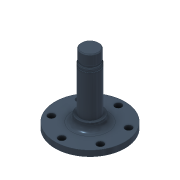
# Autodesk Inventor part: 7055-191 PART1
Saved by Autodesk Inventor 2020.1 (Build 241239000, 239)
## iProperties
Created: 2001-03-07
Part Number: 7055-191 PART1
Document SubType Name: Modeling
Designer: Joe M
Material: Steel, Mild
Engineer: Joe M
Cost Center: 6.680 kg
Authority: 849920.0 mm^3
Density: 7.86 g/cm^3
Appearance: Blue Gray (Dark/Polished)
Control State: 0
Master: False
Checked Out: False
Shininess: 20.0
Length Units: 11269
Angle Units: 11279
Time Units: 11290
Mass Units: 11283
Length Display Precision: 3
Angle Display Precision: 2
Compacted: True
SaveDate: 2003-11-30
SaveTime: 16:18
TotalMass: 6.680 kg
TotalVolume: 849920.0 mm^3
Density: 0.0
Volumn: 0.0
Area: 0.0
PropertySet Name: Model Information
Author: Joe M
Autodesk Inventor part; units mm, degrees
ref_plane "YZ Plane" through (0, 0, 0) normal (1, 0, 0) x (0, 1, 0)
ref_plane "XZ Plane" through (0, 0, 0) normal (0, 1, 0) x (-1, 0, 0)
ref_plane "XY Plane" through (0, 0, 0) normal (0, 0, 1) x (1, 0, 0)
sketch "Sketch1" plane through (-207.0981, -171.1026, -7.5) normal (0, 0, 1) x (1, 0, 0)
  circle A0 centre (207.0981, 171.1026) radius 92.5
  dimension "d40" = 185
  constraints: 1 centre point, 1 other
  measures "d40" diameter of A0
extrude "ExtrusionBlind1" add sketch "Sketch1" along normal blind 15
sketch "Sketch2" plane through (-207.0981, -171.1026, -7.5) normal (0, 0, 1) x (1, 0, 0)
  circle A0 centre (207.0981, 171.1026) radius 57.5
  circle A1 centre (207.0981, 171.1026) radius 92.5 projected
  dimension "d41" = 115
  constraints: 1 centre point, 1 concentric
  measures "d41" diameter of A0
extrude "ExtrusionBlind2" add sketch "Sketch2" against normal blind 10 contours A0
chamfer "Chamfer1" distance 2 angle 30 1 edges at (-57.5, 0, -17.5) measured on face at (-40.0277, -41.2799, -14.1667)
sketch "Sketch4" plane through (0, 0, 7.5) normal (0, 0, 1) x (1, 0, 0)
  circle A0 centre (0, 0) radius 32.5
  circle A1 centre (0, 0) radius 92.5 projected
  dimension "d42" = 65
  constraints: 1 centre point, 1 concentric
  measures "d42" diameter of A0
extrude "ExtrusionBlind3" add sketch "Sketch4" along normal blind 20 contours A0
fillet "Fillet1" radius 15 1 edges at (-32.5, 0, 7.5)
sketch "Sketch5" plane through (0, 0, 27.5) normal (0, 0, 1) x (1, 0, 0)
  circle A0 centre (0, 0) radius 25
  circle A1 centre (0, 0) radius 32.5 projected
  dimension "d43" = 50
  constraints: 3 other
  measures "d43" diameter of A0
extrude "ExtrusionBlind4" add sketch "Sketch5" along normal blind 110 contours A0
sketch "Sketch6" plane through (0, 0, 137.5) normal (0, 0, 1) x (1, 0, 0)
  circle A0 centre (0, 0) radius 23.5
  circle A1 centre (0, 0) radius 25 projected
  dimension "d44" = 47
  constraints: 3 other
  measures "d44" diameter of A0
extrude "ExtrusionBlind5" add sketch "Sketch6" along normal blind 4.15 contours A0
sketch "Sketch7" plane through (0, 0, 141.65) normal (0, 0, 1) x (1, 0, 0)
  circle A0 centre (0, 0) radius 25
  circle A1 centre (0, 0) radius 23.5 projected
  dimension "d45" = 50
  constraints: 3 other
  measures "d45" diameter of A0
extrude "ExtrusionBlind6" add sketch "Sketch7" along normal blind 4.85 contours A0 | A1
chamfer "Chamfer2" distance 2 angle 30 1 edges at (-25, 0, 146.5) measured on face at (24.9189, -2.0117, 144.8833)
sketch "Sketch8" plane through (0, 0, 146.5) normal (0, 0, 1) x (1, 0, 0)
  circle A0 centre (0, 0) radius 21.5
  circle A1 centre (0, 0) radius 23.8453 projected
  dimension "d46" = 43
  constraints: 1 centre point, 1 concentric
  measures "d46" diameter of A0
extrude "ExtrusionBlind7" add sketch "Sketch8" along normal blind 6 contours A0
sketch "Sketch9" plane through (0, 0, 152.5) normal (0, 0, 1) x (1, 0, 0)
  circle A0 centre (0, 0) radius 23.6
  circle A1 centre (0, 0) radius 21.5 projected
  dimension "d47" = 47.2
  constraints: 1 centre point, 1 concentric
  measures "d47" diameter of A0
extrude "ExtrusionBlind8" add sketch "Sketch9" along normal blind 26 contours A0 | A1
chamfer "Chamfer3" distance 2 angle 45 1 edges at (-23.6, 0, 178.5)
sketch "Sketch12" plane through (0, 0, 7.5) normal (0, 0, 1) x (1, 0, 0)
  circle A0 centre (0, 0) radius 92.5 projected
  line L0 (0, 0) -> (0, 75) construction
  dimension "d51" = 75
  constraints: 2 end point, 1 vertical
  measures "d51" distance of L0.start L0.end
hole "Hole2" at (0, 75, 7.5) direction (0, 0, -1) diameter 18 end through all clearance for "Hex Head Bolt" size "M16" standard "Ansi Metric M Profile"
pattern_circular "Circular Pattern2" count 6 over 360 about axis through (0, 0, -7.5) along (0, 0, 1) of "Hole2"
body "Solid1"
